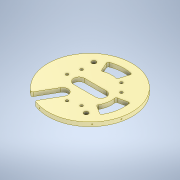
# Autodesk Inventor part: End Cap
Saved by Autodesk Inventor 2021 (Build 250183000, 183)
## iProperties
Created: 2020-11-18
Part Number: End Cap
Material: Generic
Document SubType Name: Modeling
Designer: dsouthall
Density: 1 g/cm^3
Appearance: Nylon 6
Author: dsouthall
Autodesk Inventor part; units mm, degrees
ref_plane "YZ Plane" through (0, 0, 0) normal (1, 0, 0) x (0, 1, 0)
ref_plane "XZ Plane" through (0, 0, 0) normal (0, 1, 0) x (-1, 0, 0)
ref_plane "XY Plane" through (0, 0, 0) normal (0, 0, 1) x (1, 0, 0)
sketch "Cylinders Sketch" plane through (0, 0, 0) normal (0, 1, 0) x (-1, 0, 0)
  arc A0 (34.1897, 92.0293) -> (62.6049, 75.6238) centre (0, 0) ccw
  line L0 (35.8336, 87.4656) -> (12.5214, 47.0877)
  line L1 (57.8306, 74.7656) -> (34.5185, 34.3877)
  line L2 (186.9251, 0) -> (-187.6153, 0) projected
  line L3 (49.0875, 85.022) -> (23.5199, 40.7377) construction
  arc A1 (34.5185, 34.3877) -> (34.5185, 34.3877) centre (23.5199, 40.7377) ccw
  line L4 (34.5185, 34.3877) -> (26.7764, 20.9781) construction
  line L5 (12.5214, 47.0877) -> (4.7794, 33.6781) construction
  arc A2 (12.5214, 47.0877) -> (34.5185, 34.3877) centre (23.5199, 40.7377) ccw
  arc A3 (49.0875, 85.022) -> (37.6765, 90.6577) centre (0, 0) ccw construction
  arc A4 (59.6736, 77.9577) -> (49.0875, 85.022) centre (0, 0) ccw construction
  line L6 (0, -187.5143) -> (0, 186.3188) projected
  line L7 (25.4, 0) -> (-11.3539, 0) construction
  arc A5 (25.4, -12.7) -> (25.4, 12.7) centre (25.4, 0) ccw
  arc A6 (-25.4, 12.7) -> (-25.4, -12.7) centre (-25.4, 0) ccw
  line L8 (25.4, 12.7) -> (-25.4, 12.7)
  line L9 (-25.4, -12.7) -> (25.4, -12.7)
  arc A7 (25.4, 12.7) -> (25.4, -12.7) centre (25.4, 0) ccw construction
  arc A8 (-25.4, -12.7) -> (-25.4, 12.7) centre (-25.4, 0) ccw construction
  arc A9 (62.6049, 75.6238) -> (57.8306, 74.7656) centre (60.5803, 73.1781) ccw
  arc A10 (35.8336, 87.4656) -> (34.1897, 92.0293) centre (33.084, 89.0531) ccw
  line L10 (34.5185, 34.3877) -> (34.5185, 34.3877) construction
  arc A11 (34.5185, 34.3877) -> (12.5214, 47.0877) centre (23.5199, 40.7377) ccw construction
  line L11 (12.5214, 47.0877) -> (12.5214, 47.0877) construction
  arc A12 (12.5214, 47.0877) -> (12.5214, 47.0877) centre (23.5199, 40.7377) ccw
  arc A13 (34.5185, 34.3877) -> (34.5185, 34.3877) centre (56.5155, 21.6877) ccw
  arc A14 (12.5214, 47.0877) -> (12.5214, 47.0877) centre (-9.4756, 59.7877) ccw
  dimension "d0" = 0
  dimension "d1" = 0
  dimension "d5" = 25.4
  dimension "d6" = 60
  dimension "d7" = 12.7
  dimension "d9" = 25.4
  dimension "d12" = 98.175
  dimension "d13" = 51.1351
  dimension "d14" = 60
  dimension "d15" = 25.4
  dimension "d16" = 0
  dimension "d17" = 0
  dimension "d25" = 0
  dimension "d31" = 12.7
  dimension "d32" = 50.8
  dimension "d33" = 0
  dimension "d34" = 12.7
  dimension "d35" = 25.4
  dimension "d81" = 3.175
  dimension "d168" = 25.4
  constraints: 34 point on circle, 20 end point, 15 centre point, 13 tangent, 9 parallel, 4 point on line, 3 equal radius, 2 line through centre
  measures "d0" distance of point (0, 0) A0.centre
  measures "d1" distance of point (0, 0) A0.centre
  measures "d5" distance between parallel lines of L0 L1
  measures "d6" angle of L1 L2
  measures "d7" distance from line of point (0, 0) L1
  measures "d9" distance of L4.end L5.end
  measures "d12" distance of A0.centre L3.start
  measures "d13" distance of L3.start L3.end
  measures "d14" angle of L3 L2
  measures "d15" diameter of A1
  measures "d16" distance of A1.centre L3.end
  measures "d17" distance of A1.centre L3.end
  measures "d25" distance from line of L2 L7.end
  measures "d31" radius of A5
  measures "d32" distance of A6.centre A5.centre
  measures "d33" vertical distance of A6.centre A5.centre
  measures "d34" distance between parallel lines of L2 L8
  measures "d35" distance from line of A6.centre L6
  measures "d81" radius of A9
  measures "d168" radius of A13
extrude "Cylinders Cutout" add sketch "Cylinders Sketch" along normal blind 9.525 contours A10 L0 A14 L6 A0 | L6 A14 L8 A6 L2 A0 | L2 A6 L9 L6 A0 | A14 L6 | L6 A14 | A1 A13 A5 L8 L6 A14 | L6 L9 A5 L2 A13 A0 | L1 A9 A0 L2 A13 | A13 L2 A5 | A13 L2 | A5 A13 L2
sketch "Wedges Sketch" plane through (0, 9.525, 0) normal (0, 1, 0) x (1, 0, 0)
  line L0 (0, 0) -> (-65.8567, 8.6702) construction
  arc A0 (-34.1897, -92.0293) -> (-62.6049, -75.6238) centre (0, 0) ccw construction
  line L1 (-431491.5759, 0) -> (431491.1645, 0) construction
  line L2 (0, 0) -> (-40.437, 52.6985) construction
  arc A1 (-91.0394, 11.9856) -> (-91.0394, -11.9856) centre (0, 0) ccw construction
  arc A2 (-65.8567, 8.6702) -> (-65.8567, -8.6702) centre (0, 0) ccw construction
  arc A3 (-58.4728, 70.8009) -> (-90.5518, 15.2385) centre (0, 0) ccw
  arc A4 (-42.7989, 50.799) -> (-65.3927, 11.6654) centre (0, 0) ccw
  line L3 (-55.8995, 72.8497) -> (-59.7652, 77.8875) construction
  line L4 (-42.3257, 55.1599) -> (-53.9321, 70.2857)
  line L5 (-91.0394, 11.9856) -> (-97.3351, 12.8144) construction
  line L6 (-68.9327, 9.0752) -> (-87.8352, 11.5637)
  line L7 (-60.3376, -63.8677) -> (-50.3549, -46.5772)
  line L8 (-57.8306, -74.7656) -> (-34.5185, -34.3877) construction
  line L9 (0, 0) -> (-65.8567, -8.6702) construction
  arc A5 (-90.5518, -15.2385) -> (-65.3467, -64.5108) centre (0, 0) ccw
  arc A6 (65.3927, 11.6654) -> (-40.437, 52.6985) centre (0, 0) ccw construction
  arc A7 (-65.3927, -11.6654) -> (-50.682, -42.9374) centre (0, 0) ccw
  arc A8 (90.5518, 15.2385) -> (58.4728, 70.8009) centre (0, 0) ccw construction
  line L10 (-68.9327, -9.0752) -> (-87.8352, -11.5637)
  line L11 (0, 0) -> (0, 124.9031) construction
  line L12 (431491.5759, 0) -> (-431491.1645, 0) construction
  arc A9 (90.5518, 15.2385) -> (55.8995, 72.8497) centre (0, 0) ccw
  arc A10 (65.3927, 11.6654) -> (42.7989, 50.799) centre (0, 0) ccw
  line L13 (42.3257, 55.1599) -> (53.9321, 70.2857)
  line L14 (68.9327, 9.0752) -> (87.8352, 11.5637)
  arc A11 (58.4728, -70.8009) -> (90.5518, -15.2385) centre (0, 0) ccw
  line L15 (68.9327, -9.0752) -> (87.8352, -11.5637)
  arc A12 (42.7989, -50.799) -> (65.3927, -11.6654) centre (0, 0) ccw
  line L16 (42.3257, -55.1599) -> (53.9321, -70.2857)
  arc A13 (-65.3467, -64.5108) -> (-60.3376, -63.8677) centre (-63.0872, -62.2802) ccw
  arc A14 (-50.3549, -46.5772) -> (-50.682, -42.9374) centre (-53.1045, -44.9897) ccw
  arc A15 (-65.3927, -11.6654) -> (-68.9327, -9.0752) centre (-68.5183, -12.223) ccw
  arc A16 (-87.8352, -11.5637) -> (-90.5518, -15.2385) centre (-87.4208, -14.7116) ccw
  arc A17 (-90.5518, 15.2385) -> (-87.8352, 11.5637) centre (-87.4208, 14.7116) ccw
  arc A18 (-53.9321, 70.2857) -> (-58.4728, 70.8009) centre (-56.451, 68.3528) ccw
  arc A19 (-42.7989, 50.799) -> (-42.3257, 55.1599) centre (-44.8446, 53.2271) ccw
  arc A20 (42.3257, 55.1599) -> (42.7989, 50.799) centre (44.8446, 53.2271) ccw
  arc A21 (-68.9327, 9.0752) -> (-65.3927, 11.6654) centre (-68.5183, 12.223) ccw
  arc A22 (58.4728, 70.8009) -> (53.9321, 70.2857) centre (56.451, 68.3528) ccw
  arc A23 (65.3927, 11.6654) -> (68.9327, 9.0752) centre (68.5183, 12.223) ccw
  arc A24 (65.3927, 11.6654) -> (68.9327, 9.0752) centre (68.5183, 12.223) ccw
  arc A25 (87.8352, 11.5637) -> (90.5518, 15.2385) centre (87.4208, 14.7116) ccw
  arc A26 (87.8352, 11.5637) -> (90.5518, 15.2385) centre (87.4208, 14.7116) ccw
  arc A27 (90.5518, -15.2385) -> (87.8352, -11.5637) centre (87.4208, -14.7116) ccw
  arc A28 (68.9327, -9.0752) -> (65.3927, -11.6654) centre (68.5183, -12.223) ccw
  arc A29 (42.7989, -50.799) -> (42.3257, -55.1599) centre (44.8446, -53.2271) ccw
  arc A30 (53.9321, -70.2857) -> (58.4728, -70.8009) centre (56.451, -68.3528) ccw
  point P0 (-37.8026, -90.876)
  point P1 (-59.7996, -78.176)
  point P2 (-34.6435, -34.6042)
  point P3 (91.0394, 11.9856)
  point P4 (40.437, 52.6985)
  point P5 (65.8567, 8.6702)
  point P6 (55.8995, -72.8497)
  point P7 (91.0394, -11.9856)
  point P8 (65.8567, -8.6702)
  point P9 (40.437, -52.6985)
  point P10 (58.4728, 70.8009)
  point P11 (-43.7629, -50.3996)
  dimension "d38" = 7.5
  dimension "d39" = 45
  dimension "d41" = 25.4
  dimension "d42" = 6.35
  dimension "d43" = 7.5
  dimension "d44" = 45
  dimension "d45" = 7.5
  dimension "d46" = 7.62
  dimension "d47" = 7.5
  dimension "d50" = 3.175
  constraints: 75 point on circle, 36 tangent, 30 centre point, 30 end point, 17 equal radius, 16 point on line, 10 symmetric about line, 2 concentric, 1 parallel, 1 vertical, 4 other
  measures "d38" angle of L1 L0
  measures "d39" angle of L0 L2
  measures "d41" radial gap between concentric circles of A1 A2
  measures "d42" radial gap between concentric circles of A0 A1
  measures "d43" angle of L1 L6
  measures "d44" angle of L6 L4
  measures "d45" angle of L1 L9
  measures "d46" distance between parallel lines of L8 L7
  measures "d47" angle of L1 L10
  measures "d50" radius of A13
extrude "Wedges Cutout" [suppressed]
sketch "Rope Holes Sketch" plane through (0, 9.525, 0) normal (0, 1, 0) x (1, 0, 0)
  circle A0 centre (0, 0) radius 38.1 construction
  arc A1 (-34.1897, -92.0293) -> (-62.6049, -75.6238) centre (0, 0) ccw projected
  line L0 (19.05, -32.9956) -> (-19.05, 32.9956) construction
  line L1 (-186.9251, 0) -> (187.6153, 0) construction
  circle A2 centre (-19.05, 32.9956) radius 5.08 construction
  circle A3 centre (19.05, -32.9956) radius 5.08 construction
  circle A4 centre (46.9396, -55.9404) radius 5.08
  circle A5 centre (-46.9396, 55.9404) radius 5.08
  line L2 (0, 187.5143) -> (0, -186.3188) construction
  circle A6 centre (0, 0) radius 73.025 construction
  line L3 (-46.9396, 55.9404) -> (46.9396, -55.9404) construction
  point P0 (-37.8026, -90.876)
  point P1 (-59.7996, -78.176)
  dimension "d51" = 38.1
  dimension "d52" = 60
  dimension "d53" = 0
  dimension "d54" = 0
  dimension "d55" = 0
  dimension "d56" = 0
  dimension "d57" = 10.16
  dimension "d170" = 146.05
  dimension "d173" = 40
  constraints: 6 centre point, 4 end point, 4 point on circle, 3 equal radius, 2 line through centre, 1 coincident, 1 concentric
  measures "d51" radius of A0
  measures "d52" angle of L1 L0
  measures "d53" distance of L0.end A2.centre
  measures "d54" distance of L0.end A2.centre
  measures "d55" distance of A3.centre L0.start
  measures "d56" distance of L0.start A3.centre
  measures "d57" diameter of A2
  measures "d170" diameter of A6
  measures "d173" angle of L3 L2
extrude "Rope Holes Cutout" cut sketch "Rope Holes Sketch" against normal blind 24.13
sketch "Support Holes Sketch" plane through (0, 9.525, 0) normal (0, 1, 0) x (1, 0, 0)
  circle A0 centre (0, 0) radius 53.6399 construction
  arc A1 (-34.1897, -92.0293) -> (-62.6049, -75.6238) centre (0, 0) ccw projected
  circle A2 centre (-53.6399, 0) radius 3.175
  line L0 (-186.9251, 0) -> (187.6153, 0) projected
  line L1 (0, 187.5143) -> (0, -186.3188) construction
  circle A3 centre (26.8199, -46.4535) radius 3.175
  circle A4 centre (26.8199, 46.4535) radius 3.175
  circle A5 centre (0, -53.6399) radius 3.175
  circle A6 centre (46.4535, 26.8199) radius 3.175
  circle A7 centre (-46.4535, 26.8199) radius 3.175
  point P0 (-37.8026, -90.876)
  point P1 (-59.7996, -78.176)
  dimension "d64" = 53.6399
  dimension "d66" = 0
  dimension "d67" = 53.6399
  dimension "d68" = 6.35
  dimension "d71" = 360
  dimension "d73" = 0
  dimension "d74" = 53.6399
  dimension "d77" = 360
  constraints: 7 centre point, 1 concentric, 1 equal radius, 14 other
  measures "d64" radius of A0
  measures "d66" distance from line of L0 A2.centre
  measures "d67" distance from line of L1 A2.centre
  measures "d68" diameter of A2
  measures "d73" distance from line of L1 A5.centre
  measures "d74" distance from line of L0 A5.centre
extrude "Support Holes Cutout" cut sketch "Support Holes Sketch" against normal blind 24.13 contours L0 A2 | A2 L0 | A3 | A4 | A5 | A6 | A7
sketch "Set Screw Sketch" plane through (0, 9.525, 0) normal (0, 1, 0) x (1, 0, 0)
  line L0 (-121.4507, -37.1312) -> (121.4507, 37.1312) construction
  line L1 (-37.1312, 121.4507) -> (37.1312, -121.4507) construction
  line L2 (-186.9251, 0) -> (187.6153, 0) construction
  line L3 (0, 187.5143) -> (0, -186.3188) projected
  arc A0 (-34.1897, -92.0293) -> (-62.6049, -75.6238) centre (0, 0) ccw projected
  line L4 (71.8006, -66.9552) -> (-71.8006, 66.9552) construction
  line L5 (-22.0846, -95.6588) -> (22.0846, 95.6588) construction
  line L6 (-95.6588, 22.0846) -> (95.6588, -22.0846) construction
  line L7 (-66.9552, -71.8006) -> (66.9552, 71.8006) construction
  dimension "d82" = 254
  dimension "d83" = 0
  dimension "d84" = 0
  dimension "d85" = 127
  dimension "d86" = 127
  dimension "d89" = 17
  dimension "d93" = 30
  dimension "d94" = 30
  dimension "d95" = 30
  dimension "d96" = 30
  constraints: 12 end point, 2 coincident, 2 perpendicular, 13 other
  measures "d82" distance of L0.start L0.end
  measures "d83" distance from line of L0 point (0, 0)
  measures "d84" distance from line of point (0, 0) L1
  measures "d85" distance of point (0, 0) L0.start
  measures "d86" distance of point (0, 0) L1.start
  measures "d89" angle of L3 L1
  measures "d93" angle of L1 L4
  measures "d94" angle of L1 L5
  measures "d95" angle of L7 L0
  measures "d96" angle of L0 L6
ref_plane "Edge Hole Plane 1" through (71.8006, 9.525, 66.9552) normal (0.7313537, 0, 0.6819984) x (0, 1, 0)
ref_plane "Edge Hole Plane 2" through (-22.0846, 9.525, 95.6588) normal (-0.2249511, 0, 0.9743701) x (0, -1, 0)
sketch "Edge Hole Center 1" plane through (71.8006, 9.525, 66.9552) normal (0.7313537, 0, 0.6819984) x (0, 1, 0)
  line L0 (0, -98.175) -> (0, 98.175) projected
  point P0 (-9.525, 0)
  point P1 (-4.7625, 0)
  point P2 (0, 90.6233)
  point P3 (0, 98.0042)
  dimension "d97" = 4.7625
  dimension "d98" = 0
  measures "d97" distance from line of L0 point (-4.763, 0)
  measures "d98" vertical distance of point (-9.525, 0) point (-4.763, 0)
sketch "Edge Hole Center 2" plane through (-22.0846, 9.525, 95.6588) normal (-0.2249511, 0, 0.9743701) x (0, -1, 0)
  line L0 (0, 98.175) -> (0, -98.175) projected
  line L1 (9.525, 98.175) -> (9.525, -98.175) projected
  point P0 (9.525, 0)
  point P1 (4.7625, 0)
  point P2 (0, -12.6113)
  point P3 (0, -43.9887)
  point P4 (9.525, -12.6113)
  point P5 (9.525, -43.9887)
  dimension "d100" = 0
  dimension "d167" = 4.7625
  measures "d100" vertical distance of point (9.525, 0) point (4.763, 0)
  measures "d167" distance from line of point (4.763, 0) L1
ref_plane "Central Plane" through (0, 4.7625, 0) normal (0, 1, 0) x (1, 0, 0)
hole "Insert Edge Hole 1" [suppressed]
hole "Insert Edge Hole 2" [suppressed]
pattern_circular "Circular Pattern2" [suppressed]
hole "4-40 2" at (-22.0846, 4.7625, 95.6588) direction (0.2249511, 0, -0.9743701) diameter 2.1565 depth 8.8646 tip angle 118 thread size "4-40 UNC" class "2B" standard "ANSI Unified Screw Threads"
hole "4-40 1" at (71.8006, 4.7625, 66.9552) direction (-0.7313537, 0, -0.6819984) diameter 2.1565 depth 8.8646 tip angle 118 thread size "4-40 UNC" class "2B" standard "ANSI Unified Screw Threads"
pattern_circular "Circular Pattern3" count 4 over 360 about axis through (0, -10, 0) along (0, 1, 0) of "4-40 2", "4-40 1"
sketch "Cutouts" plane through (0, 9.525, 0) normal (0, 1, 0) x (1, 0, 0)
  arc A0 (-34.1897, -92.0293) -> (-62.6049, -75.6238) centre (0, 0) ccw projected
  line L0 (-85.022, 49.0875) -> (85.022, -49.0875) construction
  line L1 (-12.5214, -47.0877) -> (-35.8336, -87.4656) projected
  line L2 (49.0875, 85.022) -> (-49.0875, -85.022) construction
  arc A1 (66.3598, -43.0946) -> (77.3959, 16.451) centre (0, 0) ccw
  arc A2 (42.6045, -27.6677) -> (49.6899, 10.5619) centre (0, 0) ccw
  line L3 (21.1411, 86.7788) -> (19.0399, 87.2639) projected
  arc A3 (14.0024, 48.8321) -> (-20.6622, 46.4081) centre (0, 0) ccw
  arc A4 (21.8098, 76.0598) -> (-32.183, 72.2843) centre (0, 0) ccw
  line L4 (66.3598, -43.0946) -> (42.6045, -27.6677)
  line L5 (77.3959, 16.451) -> (49.6899, 10.5619)
  line L6 (14.0024, 48.8321) -> (21.8098, 76.0598)
  line L7 (-20.6622, 46.4081) -> (-32.183, 72.2843)
  dimension "d185" = 50.8
  dimension "d188" = 50.8
  dimension "d189" = 45
  dimension "d190" = 3
  dimension "d191" = 40
  dimension "d192" = 14
  dimension "d193" = 19.05
  dimension "d194" = 19.05
  constraints: 14 point on circle, 12 end point, 10 line through centre, 4 centre point, 3 coincident, 2 perpendicular
  measures "d185" radius of A3
  measures "d188" radius of A2
  measures "d189" angle of L4 L5
  measures "d190" angle of L0 L4
  measures "d191" angle of L7 L6
  measures "d192" angle of L2 L6
  measures "d193" radial gap between concentric circles of A4 A0
  measures "d194" radial gap between concentric circles of A1 A0
extrude "Cutouts extrude" cut sketch "Cutouts" against normal blind 25.4
fillet "Fillet1" radius 3.175 8 edges at (77.3959, 4.7625, -16.451) (66.3598, 4.7625, 43.0946) (42.6045, 4.7625, 27.6677) (49.6899, 4.7625, -10.5619) (14.0024, 4.7625, -48.8321) (-20.6622, 4.7625, -46.4081) (-32.183, 4.7625, -72.2843) (21.8098, 4.7625, -76.0598)
sketch "Edge Hole Center 1 - Unthreaded" plane through (71.8006, 9.525, 66.9552) normal (0.7313537, 0, 0.6819984) x (0, 1, 0)
  line L0 (0, -98.175) -> (0, 98.175) projected
  point P0 (-9.525, 0)
  point P1 (-4.7625, 0)
  point P2 (0, 90.6233)
  point P3 (0, 98.0042)
  dimension "d198" = 4.7625
  dimension "d199" = 0
  measures "d198" distance from line of point (-4.763, 0) L0
  measures "d199" vertical distance of point (-9.525, 0) point (-4.763, 0)
sketch "Edge Hole Center 2 - Unthreaded" plane through (-22.0846, 9.525, 95.6588) normal (-0.2249511, 0, 0.9743701) x (0, -1, 0)
  line L0 (0, 98.175) -> (0, -98.175) projected
  point P0 (9.525, 0)
  point P1 (4.7625, 0)
  point P2 (0, -12.6113)
  point P3 (0, -43.9887)
  dimension "d200" = 4.7625
  dimension "d201" = 0
  measures "d200" distance from line of point (4.763, 0) L0
  measures "d201" vertical distance of point (9.525, 0) point (4.763, 0)
hole "Edge Hole 1 - Unthreaded" [suppressed]
hole "Edge Hole 2 - Unthreaded" [suppressed]
pattern_circular "Circular Pattern4" [suppressed]
equation "\"d7\" = 0.5 * d5"
body "Solid1"
